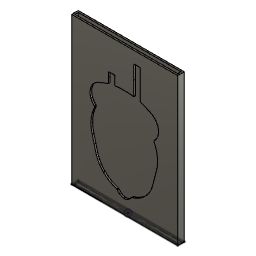
DIYCard Holder (Autodesk Fusion 360 design; units mm, degrees)
Autodesk Fusion 360 part; units mm, degrees
note: some values were not read from the file. Set by a fixed rule: which sketch regions a step uses.
sketch "Sketch1" plane through (0, 0, 0) normal (0, 1, 0) x (1, 0, 0)
  line L0 (32, 1.05) -> (-32, 1.05)
  line L1 (-32, 1.05) -> (-32, -1.05)
  line L2 (-32, -1.05) -> (32, -1.05)
  line L3 (32, -1.05) -> (32, 1.05)
  line L4 (32, 1.05) -> (-32, -1.05) construction
  line L5 (-32, 1.05) -> (32, -1.05) construction
  line L6 (-33, -2.05) -> (33, -2.05)
  line L7 (33, -2.05) -> (33, 2.05)
  line L8 (33, 2.05) -> (-33, 2.05)
  line L9 (-33, 2.05) -> (-33, -2.05)
  dimension "d1" = 64
  dimension "d2" = 2.1
  dimension "d16" = 1
  dimension "d17" = 1
  dimension "d18" = 1
  dimension "d19" = 1
  constraint horizontal L0
  constraint perpendicular L0 L1
  constraint parallel L0 L2
  constraint parallel L1 L3
  constraint coincident L4 origin
  constraint coincident L5 origin
  constraint parallel L2 L6
  constraint parallel L3 L7
  constraint parallel L0 L8
  constraint parallel L1 L9
  measures "d1" distance of L1.end L2.end
  measures "d2" distance of L0.end L1.end
  measures "d16" distance of L0 L8
  measures "d17" distance of L2 L6
  measures "d18" distance of L1 L9
  measures "d19" distance of L3 L7
extrude "Extrude1" add sketch "Sketch1" along normal blind 1.5 contours L0 L1 L2 L3 | L6 L7 L8 L9
extrude "Extrude2" add sketch "Sketch1" along normal blind 90 from surface at 1.5
sketch "fullAcorn" plane through (-108.5, 177.5, 2.05) normal (0, 0, 1) x (1, 0, 0)
  spline S0 degree 3 poles (126.9984, -128.196) (128.375, -126.8389) (129.2314, -125.1119) (129.485, -123.1813) (129.5543, -122.6542) (129.5439, -121.5132) (129.4647, -120.9902) knots 0 0 0 0 1 1 1 2 2 2 2
  ellipse E0 centre (110.9773, -128.8447) end of major axis (128.1231, -117.446) minor radius 13.0294 (129.4647, -120.9902) -> (125.6655, -115.0219) ccw
  spline S1 degree 3 poles (125.6655, -115.0219) (125.0195, -114.5958) (124.5237, -114.3667) (122.5228, -113.5691) knots 3 3 3 3 4 4 4 4
  spline S2 degree 3 poles (122.5228, -113.5691) (120.1502, -112.6231) (119.9514, -112.5476) (118.9765, -112.2259) knots 4 4 4 4 5 5 5 5
  line L0 (118.9765, -112.2259) -> (118.1396, -111.9496)
  line L1 (118.1396, -111.9496) -> (118.1176, -102.7484)
  line L2 (118.1176, -102.7484) -> (118.0955, -93.5476)
  line L3 (118.0955, -93.5476) -> (117.8695, -93.4728)
  spline S3 degree 3 poles (117.8695, -93.4728) (117.2077, -93.253) (115.0032, -93.2699) (114.3397, -93.4994) knots 9 9 9 9 10 10 10 10
  line L4 (114.3397, -93.4994) -> (114.1747, -93.5569)
  line L5 (114.1747, -93.5569) -> (114.1636, -102.3123)
  line L6 (114.1636, -102.3123) -> (114.1526, -111.0673)
  line L7 (114.1526, -111.0673) -> (113.9873, -111.0411)
  spline S4 degree 3 poles (113.9873, -111.0411) (113.3038, -110.9329) (111.863, -110.7889) (110.8484, -110.7273) (109.3567, -110.6366) (106.2554, -110.6587) (104.9015, -110.7696) knots 14 14 14 14 15 15 15 16 16 16 16
  spline S5 degree 3 poles (104.9015, -110.7696) (104.1291, -110.833) (102.8648, -110.9767) (102.4892, -111.0439) knots 16 16 16 16 17 17 17 17
  line L8 (102.4892, -111.0439) -> (102.3459, -111.0694)
  line L9 (102.3459, -111.0694) -> (102.3459, -108.3343)
  line L10 (102.3459, -108.3343) -> (102.3459, -105.5989)
  line L11 (102.3459, -105.5989) -> (102.2467, -105.5355)
  spline S6 degree 3 poles (102.2467, -105.5355) (102.1923, -105.5004) (101.9642, -105.4501) (101.7403, -105.4232) knots 21 21 21 21 22 22 22 22
  spline S7 degree 3 poles (101.7403, -105.4232) (101.2339, -105.3629) (99.3597, -105.3601) (98.8974, -105.419) knots 22 22 22 22 23 23 23 23
  spline S8 degree 3 poles (98.8974, -105.419) (98.3165, -105.4931) (98.3834, -105.0718) (98.3703, -108.7498) knots 23 23 23 23 24 24 24 24
  line L12 (98.3703, -108.7498) -> (98.3593, -111.9441)
  line L13 (98.3593, -111.9441) -> (97.456, -112.2452)
  spline S9 degree 3 poles (97.456, -112.2452) (96.4521, -112.58) (95.905, -112.7881) (93.6236, -113.7024) (91.5779, -114.5224) (91.0598, -114.7897) (90.1648, -115.4887) knots 26 26 26 26 27 27 27 28 28 28 28
  ellipse E1 centre (89.2579, -116.6357) end of major axis (88.0374, -117.9466) minor radius 0.2027 (90.1648, -115.4887) -> (89.5274, -116.0659) ccw
  line L14 (89.5274, -116.0659) -> (89.5265, -116.0659)
  line L15 (89.5265, -116.0659) -> (89.5265, -116.0668)
  ellipse E2 centre (89.5267, -116.313) end of major axis (88.4706, -117.3898) minor radius 0.1737 (89.5265, -116.0668) -> (88.6579, -117.0332) ccw
  spline S10 degree 3 poles (88.6579, -117.0332) (86.8706, -119.39) (86.4461, -122.5229) (87.543, -125.2676) knots 32 32 32 32 33 33 33 33
  spline S11 degree 3 poles (87.543, -125.2676) (87.9868, -126.3783) (88.6338, -127.3416) (89.526, -128.2173) knots 33 33 33 33 34 34 34 34
  line L16 (89.526, -128.2173) -> (89.5844, -128.2747)
  line L17 (89.5844, -128.2747) -> (89.9231, -128.6428)
  line L18 (89.9231, -128.6428) -> (89.926, -128.6593)
  line L19 (89.926, -128.6593) -> (89.7794, -129.0579)
  line L20 (89.7794, -129.0579) -> (89.6211, -129.3852)
  spline S12 degree 3 poles (89.6211, -129.3852) (89.0658, -130.5317) (88.735, -131.3692) (88.4112, -132.4483) knots 40 40 40 40 41 41 41 41
  spline S13 degree 3 poles (88.4112, -132.4483) (87.7993, -134.4877) (87.5375, -136.2985) (87.5375, -138.4834) (87.5375, -140.4781) (87.7442, -141.9719) (88.3306, -144.2105) knots 41 41 41 41 42 42 42 43 43 43 43
  spline S14 degree 3 poles (88.3306, -144.2105) (88.4512, -144.6715) (88.9893, -146.7726) (89.5253, -148.8807) knots 43 43 43 43 44 44 44 44
  spline S15 degree 3 poles (89.5253, -148.8807) (90.0621, -150.9887) (90.5789, -152.9841) (90.6739, -153.3145) (91.529, -156.2856) (93.0359, -158.8656) (95.2056, -161.0767) knots 44 44 44 44 45 45 45 46 46 46 46
  spline S16 degree 3 poles (95.2056, -161.0767) (97.5352, -163.451) (100.2975, -165.0558) (103.6289, -165.9715) knots 46 46 46 46 47 47 47 47
  spline S17 degree 3 poles (103.6289, -165.9715) (103.8397, -166.0293) (103.8859, -166.0607) (103.9362, -166.183) knots 47 47 47 47 48 48 48 48
  spline S18 degree 3 poles (103.9362, -166.183) (104.1436, -166.686) (104.8898, -167.5469) (105.4727, -167.9565) knots 48 48 48 48 49 49 49 49
  ellipse E3 centre (107.6789, -166.0654) end of major axis (111.237, -167.0515) minor radius 2.6842 (105.4727, -167.9565) -> (108.029, -168.8271) ccw
  ellipse E4 centre (109.0371, -166.3569) end of major axis (112.2951, -165.2452) minor radius 2.3377 (108.029, -168.8271) -> (110.4199, -168.3066) ccw
  spline S19 degree 3 poles (110.4199, -168.3066) (111.3156, -167.8573) (111.9815, -167.199) (112.5362, -166.2126) knots 51 51 51 51 52 52 52 52
  spline S20 degree 3 poles (112.5362, -166.2126) (112.6409, -166.0262) (112.6685, -166.0069) (112.9055, -165.9542) knots 52 52 52 52 53 53 53 53
  spline S21 degree 3 poles (112.9055, -165.9542) (113.3172, -165.8633) (114.658, -165.4099) (115.2416, -165.1653) knots 53 53 53 53 54 54 54 54
  spline S22 degree 3 poles (115.2416, -165.1653) (117.5257, -164.2062) (119.4209, -162.9356) (121.16, -161.1966) (122.6317, -159.7248) (123.6983, -158.2406) (124.6237, -156.3776) (125.3578, -154.8996) (125.6468, -154.0438) (126.3727, -151.1934) knots 54 54 54 54 55 55 55 56 56 56 57 57 57 57
  spline S23 degree 3 poles (126.3727, -151.1934) (126.5546, -150.4789) (127.0838, -148.407) (127.5482, -146.5897) (128.4578, -143.0302) (128.5993, -142.4225) (128.7361, -141.504) knots 57 57 57 57 58 58 58 59 59 59 59
  spline S24 degree 3 poles (128.7361, -141.504) (129.3055, -137.6738) (128.7815, -133.7147) (127.235, -130.1569) knots 59 59 59 59 60 60 60 60
  spline S25 degree 3 poles (127.235, -130.1569) (127.0142, -129.6481) (126.5884, -128.7699) (126.5632, -128.7699) (126.5615, -128.7699) (126.5536, -128.773) (126.5422, -128.778) knots 60 60 60 60 61 61 61 62 62 62 62
  ellipse E5 centre (126.0019, -128.046) end of major axis (125.3918, -129.1069) minor radius 0.8731 (126.5422, -128.778) -> (126.8134, -128.3784) ccw
  line L21 (126.8134, -128.3784) -> (126.9984, -128.196)
extrude "Extrude5" cut sketch "fullAcorn" against normal up to surface (3.1 mm away)
sketch "acornBottom" plane through (-108, 186.5, 1.675) normal (0, 0, 1) x (1, 0, 0)
  spline S0 degree 3 poles (90.3212, -162.1673) (91.1762, -165.1383) (92.6831, -167.7184) (94.8528, -169.9294) knots 0 0 0 0 1 1 1 1
  spline S1 degree 3 poles (94.8528, -169.9294) (97.1824, -172.3038) (99.9447, -173.9085) (103.2761, -174.8242) knots 1 1 1 1 2 2 2 2
  spline S2 degree 3 poles (103.2761, -174.8242) (103.4869, -174.8821) (103.5331, -174.9135) (103.5834, -175.0358) knots 2 2 2 2 3 3 3 3
  spline S3 degree 3 poles (103.5834, -175.0358) (103.7908, -175.5388) (104.537, -176.3997) (105.1199, -176.8093) knots 3 3 3 3 4 4 4 4
  ellipse E0 centre (107.3261, -174.9182) end of major axis (110.8842, -175.9043) minor radius 2.6842 (105.1199, -176.8093) -> (107.6762, -177.6799) ccw
  ellipse E1 centre (108.6843, -175.2096) end of major axis (111.9423, -174.098) minor radius 2.3377 (107.6762, -177.6799) -> (110.0671, -177.1593) ccw
  spline S4 degree 3 poles (110.0671, -177.1593) (110.9628, -176.7101) (111.6287, -176.0517) (112.1834, -175.0654) knots 6 6 6 6 7 7 7 7
  spline S5 degree 3 poles (112.1834, -175.0654) (112.2881, -174.879) (112.3157, -174.8597) (112.5527, -174.807) knots 7 7 7 7 8 8 8 8
  spline S6 degree 3 poles (112.5527, -174.807) (112.9644, -174.7161) (114.3052, -174.2627) (114.8888, -174.0181) knots 8 8 8 8 9 9 9 9
  spline S7 degree 3 poles (114.8888, -174.0181) (117.1729, -173.059) (119.0681, -171.7884) (120.8072, -170.0493) (122.2789, -168.5776) (123.3455, -167.0934) (124.2709, -165.2303) knots 9 9 9 9 10 10 10 11 11 11 11
  spline S8 degree 3 poles (124.2709, -165.2303) (125.005, -163.7524) (125.2941, -162.8966) (126.02, -160.0462) knots 11 11 11 11 12 12 12 12
  spline S9 degree 3 poles (126.02, -160.0462) (126.0248, -160.0279) (126.0306, -160.0048) (126.0355, -159.9848) knots 12 12 12 12 13 13 13 13
  line L0 (126.0355, -159.9848) -> (89.7491, -159.9848)
  spline S10 degree 3 poles (89.7491, -159.9848) (90.0388, -161.1086) (90.2619, -161.9613) (90.3212, -162.1673) knots 14 14 14 14 15 15 15 15
extrude "Extrude4" [suppressed]
extrude "Extrude3" [suppressed]
